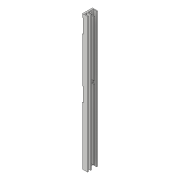
# Autodesk Inventor part: 6089-111_FF_right_heatsink
Saved by Autodesk Inventor 2017.3 (Build 213256000, 256)
## iProperties
Created: 2019-03-02
Part Number: 6089-111_FF_right_heatsink
Material: Generic
Document SubType Name: Modeling
Designer: crs5
Density: 1 g/cm^3
Appearance: Default
Author: crs5
Autodesk Inventor part; units mm, degrees
ref_plane "YZ Plane" through (0, 0, 0) normal (1, 0, 0) x (0, 1, 0)
ref_plane "XZ Plane" through (0, 0, 0) normal (0, 1, 0) x (-1, 0, 0)
ref_plane "XY Plane" through (0, 0, 0) normal (0, 0, 1) x (1, 0, 0)
sketch "Sketch1" plane through (0, 0, 0) normal (0, 1, 0) x (-1, 0, 0)
  line L0 (0, 0) -> (9.91, 0)
  line L1 (9.91, 0) -> (9.91, -19.22)
  line L2 (9.91, -19.22) -> (0, -19.22)
  line L3 (0, -19.22) -> (0, 0)
  dimension "d0" = 19.22
  dimension "d1" = 9.91
  constraints: 8 end point, 2 parallel, 1 horizontal, 1 perpendicular
  measures "d0" distance of L2.end L0.start
  measures "d1" distance of L0.start L0.end
extrude "Extrusion1" add sketch "Sketch1" along normal blind 258.6
sketch "Sketch2" plane through (0, 0, 0) normal (0, -1, 0) x (1, 0, 0)
  line L0 (0, -1.7) -> (-7, -1.7)
  line L1 (-7, -1.7) -> (-7, -5.84)
  line L2 (-7, -5.84) -> (0, -5.84)
  line L3 (0, -5.84) -> (0, -1.7)
  line L4 (0, 0) -> (-9.91, 0) projected
  line L5 (0, -19.22) -> (0, 0) projected
  dimension "d31" = 1.7
  dimension "d32" = 4.14
  dimension "d33" = 7
  constraints: 8 end point, 2 parallel, 1 collinear, 1 horizontal, 1 perpendicular
  measures "d31" distance between parallel lines of L0 L4
  measures "d32" distance between parallel lines of L2 L0
  measures "d33" distance of L0.start L0.end
extrude "Extrusion2" cut sketch "Sketch2" against normal through all
sketch "Sketch3" plane through (0, 0, 0) normal (0, -1, 0) x (1, 0, 0)
  line L0 (0, -7.54) -> (-7, -7.54)
  line L1 (-7, -7.54) -> (-7, -11.68)
  line L2 (-7, -11.68) -> (0, -11.68)
  line L3 (0, -11.68) -> (0, -7.54)
  line L4 (0, -5.84) -> (-7, -5.84) projected
  line L5 (-7, -5.84) -> (-7, -1.7) projected
  point P0 (0, 0)
  dimension "d39" = 1.7
  dimension "d40" = 4.14
  constraints: 8 end point, 2 parallel, 1 collinear, 1 horizontal, 1 perpendicular
  measures "d39" distance between parallel lines of L0 L4
  measures "d40" distance between parallel lines of L2 L0
extrude "Extrusion3" cut sketch "Sketch3" against normal through all
sketch "Sketch4" plane through (0, 0, 0) normal (0, -1, 0) x (1, 0, 0)
  line L0 (0, -13.38) -> (-7, -13.38)
  line L1 (-7, -13.38) -> (-7, -17.52)
  line L2 (-7, -17.52) -> (0, -17.52)
  line L3 (0, -17.52) -> (0, -13.38)
  line L4 (0, -11.68) -> (-7, -11.68) projected
  line L5 (-7, -11.68) -> (-7, -7.54) projected
  point P0 (0, 0)
  dimension "d43" = 1.7
  dimension "d44" = 4.14
  constraints: 8 end point, 2 parallel, 1 collinear, 1 horizontal, 1 perpendicular
  measures "d43" distance between parallel lines of L0 L4
  measures "d44" distance between parallel lines of L2 L0
extrude "Extrusion4" cut sketch "Sketch4" against normal through all
hole "Hole7" at (0, 3, -12.53) direction (-1, 0, 0) diameter 2.9 end through all counterbore diameter 6.5 counterbore depth 7 clearance for "Socket Head Cap Screw" size "M2.5" standard "Ansi Metric M Profile"
hole "Hole8" at (0, 143.4, -12.53) direction (-1, 0, 0) diameter 2.9 end through all counterbore diameter 6.5 counterbore depth 7 clearance for "Socket Head Cap Screw" size "M2.5" standard "Ansi Metric M Profile"
hole "Hole15" at (0, 255.6, -12.53) direction (-1, 0, 0) diameter 2.9 end through all counterbore diameter 6.5 counterbore depth 7
sketch "Sketch6" plane through (-9.91, 0, -19.22) normal (-1, 0, 0) x (0, 0, 1)
  line L0 (0, 0) -> (0, 258.6) projected
  line L1 (19.22, 0) -> (19.22, 258.6) projected
  line L2 (0, 138.6) -> (19.22, 138.6)
  line L3 (19.22, 138.6) -> (19.22, 111.2)
  line L4 (19.22, 111.2) -> (0, 111.2)
  line L5 (0, 111.2) -> (0, 138.6)
  line L6 (19.22, 0) -> (0, 0) projected
  dimension "d158" = 111.2
  dimension "d159" = 138.6
  constraints: 8 end point, 2 parallel, 2 point on line, 1 horizontal, 1 perpendicular
  measures "d158" distance between parallel lines of L4 L6
  measures "d159" distance between parallel lines of L2 L6
extrude "Extrusion6" cut sketch "Sketch6" against normal blind 1.45 contours L0 L2 L1 L4
sketch "Sketch7" plane through (-9.91, 258.6, -19.22) normal (-1, 0, 0) x (0, 0, 1)
  line L0 (0, -120) -> (0, 0) projected
  line L1 (19.22, -120) -> (19.22, 0) projected
  line L2 (0, -6.2) -> (19.22, -6.2)
  line L3 (19.22, -6.2) -> (19.22, -33.6)
  line L4 (19.22, -33.6) -> (0, -33.6)
  line L5 (0, -33.6) -> (0, -6.2)
  line L6 (19.22, -258.6) -> (0, -258.6) projected
  dimension "d162" = 225
  dimension "d163" = 252.4
  constraints: 8 end point, 2 parallel, 2 point on line, 1 horizontal, 1 perpendicular
  measures "d162" distance between parallel lines of L4 L6
  measures "d163" distance between parallel lines of L2 L6
extrude "Extrusion7" cut sketch "Sketch7" against normal blind 1.45
body "Solid1"
